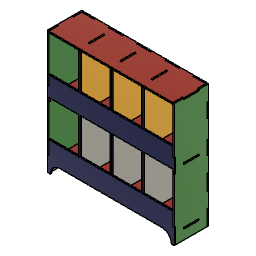
sorted_smarties_collector_finger_joints (Autodesk Fusion 360 design; units mm, degrees)
Autodesk Fusion 360 part; units mm, degrees
note: some values were not read from the file. Chosen so that the rebuilt part matches the saved one: which bodies a step acts on; which face or edge a step refers to; that a step has no effect. Set by a fixed rule: which sketch regions a step uses.
(part 1 of 2)
sketch "Sorted Smarties Collector" plane through (0, 0, 0) normal (0, 1, 0) x (1, 0, 0)
  line L0 (0, 0) -> (266, 0)
  line L1 (266, 0) -> (266, -258)
  line L2 (266, -258) -> (0, -258)
  line L3 (0, -258) -> (0, 0)
  dimension "d1" = 266
  dimension "d41" = 258
  constraint horizontal L0
  constraint vertical L1
  constraint horizontal L2
  constraint vertical L3
  constraint coincident L0.start L3.end
  measures "d1" distance of L0.start L0.end
  measures "d41" distance of L0.end L1.end
extrude "Extrude1" add sketch "Sorted Smarties Collector" along normal blind 3 makes body 1
sketch "Smartie Collectors" plane through (0, 3, 0) normal (0, 1, 0) x (-1, 0, 0)
  line L0 (0, 258) -> (-266, 258)
  line L1 (-266, 258) -> (-266, 0)
  line L2 (-266, 0) -> (0, 0)
  line L3 (0, 0) -> (0, 258)
  line L4 (-263, 255) -> (-200.25, 255)
  line L5 (-200.25, 255) -> (-200.25, 140.5)
  line L6 (-200.25, 140.5) -> (-263, 140.5)
  line L7 (-263, 140.5) -> (-263, 255)
  line L8 (-197.25, 255) -> (-134.5, 255)
  line L9 (-134.5, 255) -> (-134.5, 140.5)
  line L10 (-134.5, 140.5) -> (-197.25, 140.5)
  line L11 (-197.25, 140.5) -> (-197.25, 255)
  line L12 (-131.5, 255) -> (-68.75, 255)
  line L13 (-68.75, 255) -> (-68.75, 140.5)
  line L14 (-68.75, 140.5) -> (-131.5, 140.5)
  line L15 (-131.5, 140.5) -> (-131.5, 255)
  line L16 (-65.75, 255) -> (-3, 255)
  line L17 (-3, 255) -> (-3, 140.5)
  line L18 (-3, 140.5) -> (-65.75, 140.5)
  line L19 (-65.75, 140.5) -> (-65.75, 255)
  line L20 (-263, 137.5) -> (-200.25, 137.5)
  line L21 (-200.25, 137.5) -> (-200.25, 23)
  line L22 (-200.25, 23) -> (-263, 23)
  line L23 (-263, 23) -> (-263, 137.5)
  line L24 (-197.25, 137.5) -> (-134.5, 137.5)
  line L25 (-134.5, 137.5) -> (-134.5, 23)
  line L26 (-134.5, 23) -> (-197.25, 23)
  line L27 (-197.25, 23) -> (-197.25, 137.5)
  line L28 (-131.5, 137.5) -> (-68.75, 137.5)
  line L29 (-68.75, 137.5) -> (-68.75, 23)
  line L30 (-68.75, 23) -> (-131.5, 23)
  line L31 (-131.5, 23) -> (-131.5, 137.5)
  line L32 (-65.75, 137.5) -> (-3, 137.5)
  line L33 (-3, 137.5) -> (-3, 23)
  line L34 (-3, 23) -> (-65.75, 23)
  line L35 (-65.75, 23) -> (-65.75, 137.5)
  line L36 (-263, 0) -> (-3, 0)
  line L37 (-3, 0) -> (-3, 20)
  line L38 (-3, 20) -> (-263, 20)
  line L39 (-263, 20) -> (-263, 0)
  dimension "d51" = 3
  dimension "d52" = 3
  dimension "d53" = 3
  dimension "d54" = 20
  dimension "d55" = 3
  dimension "d56" = 3
  dimension "d57" = 3
  dimension "d58" = 3
  dimension "d59" = 3
  dimension "d60" = 114.5
  dimension "d61" = 114.5
  dimension "d62" = 62.75
  dimension "d63" = 62.75
  dimension "d64" = 62.75
  dimension "d65" = 62.75
  constraint horizontal L4
  constraint vertical L5
  constraint horizontal L6
  constraint vertical L7
  constraint horizontal L8
  constraint vertical L9
  constraint horizontal L10
  constraint vertical L11
  constraint horizontal L12
  constraint vertical L13
  constraint horizontal L14
  constraint vertical L15
  constraint horizontal L16
  constraint vertical L17
  constraint horizontal L18
  constraint vertical L19
  constraint horizontal L20
  constraint vertical L21
  constraint horizontal L22
  constraint vertical L23
  constraint horizontal L24
  constraint vertical L25
  constraint horizontal L26
  constraint vertical L27
  constraint horizontal L28
  constraint vertical L29
  constraint horizontal L30
  constraint vertical L31
  constraint horizontal L32
  constraint vertical L33
  constraint horizontal L34
  constraint vertical L35
  constraint collinear L4 L8
  constraint collinear L8 L12
  constraint collinear L12 L16
  constraint collinear L6 L10
  constraint collinear L10 L14
  constraint collinear L14 L18
  constraint collinear L22 L26
  constraint collinear L26 L30
  constraint collinear L30 L34
  constraint collinear L20 L24
  constraint collinear L24 L28
  constraint collinear L28 L32
  constraint horizontal L36
  constraint vertical L37
  constraint horizontal L38
  constraint vertical L39
  constraint coincident L2 L36.start
  constraint collinear L23 L39
  constraint collinear L7 L23
  constraint collinear L5 L21
  constraint collinear L11 L27
  constraint collinear L9 L25
  constraint collinear L15 L31
  constraint collinear L13 L29
  constraint collinear L19 L35
  constraint collinear L17 L33
  constraint collinear L33 L37
  measures "d51" distance of L0 L4
  measures "d52" distance of L6 L20
  measures "d53" distance of L22 L38
  measures "d54" distance of L36 L38
  measures "d55" distance of L5 L11
  measures "d56" distance of L9 L15
  measures "d57" distance of L13 L19
  measures "d58" distance of L1 L7
  measures "d59" distance of L3 L17
  measures "d60" distance of L16.end L17.end
  measures "d61" distance of L32.end L33.end
  measures "d62" distance of L4.start L4.end
  measures "d63" distance of L8.start L8.end
  measures "d64" distance of L12.start L12.end
  measures "d65" distance of L16.start L16.end
extrude "Extrude2" add sketch "Smartie Collectors" along normal blind 69 contours L0 L1 L2 L3 L37 L38 L39 bodies 1
sketch "Front Panel" plane through (266, 0, 0) normal (1, 0, 0) x (0, 1, 0)
  line L0 (0, 258) -> (0, 0)
  line L1 (0, 0) -> (72, 0)
  line L2 (72, 0) -> (72, 258)
  line L3 (72, 258) -> (0, 258)
  line L4 (72, 258) -> (69, 258)
  line L5 (69, 258) -> (69, 0)
  line L6 (69, 0) -> (72, 0)
  line L7 (72, 0) -> (72, 258)
  dimension "d66" = 3
  constraint horizontal L4
  constraint vertical L5
  constraint horizontal L6
  constraint vertical L7
  constraint coincident L1 L5.end
  constraint coincident L2.end L3.start
  measures "d66" distance of L5.end L1.end
extrude "Extrude3" add sketch "Front Panel" against normal blind 266 contours L1 L2 L3 L4 L5 L6 L7 bodies 1
sketch "Front Openings" plane through (0, 72, 0) normal (0, 1, 0) x (-1, 0, 0)
  line L0 (-266, 0) -> (0, 0)
  line L1 (0, 0) -> (0, 258)
  line L2 (0, 258) -> (-266, 258)
  line L3 (-266, 258) -> (-266, 0)
  line L4 (0, 258) -> (-266, 258)
  line L5 (-197.25, 255) -> (-134.5, 255)
  line L6 (-263, 255) -> (-200.25, 255)
  line L7 (-200.25, 140.5) -> (-263, 140.5)
  line L8 (-263, 137.5) -> (-200.25, 137.5)
  line L9 (-200.25, 23) -> (-263, 23)
  line L10 (-134.5, 23) -> (-197.25, 23)
  line L11 (-68.75, 23) -> (-131.5, 23)
  line L12 (-3, 23) -> (-65.75, 23)
  line L13 (-131.5, 137.5) -> (-68.75, 137.5)
  line L14 (-197.25, 137.5) -> (-134.5, 137.5)
  line L15 (-134.5, 140.5) -> (-197.25, 140.5)
  line L16 (-68.75, 140.5) -> (-131.5, 140.5)
  line L17 (-3, 140.5) -> (-65.75, 140.5)
  line L18 (-65.75, 137.5) -> (-3, 137.5)
  line L19 (-131.5, 255) -> (-68.75, 255)
  line L20 (-65.75, 255) -> (-3, 255)
  line L21 (-3, 20) -> (-263, 20)
  line L22 (-3, 0) -> (-3, 20)
  line L23 (-263, 20) -> (-263, 0)
  line L24 (-263, 23) -> (-263, 137.5)
  line L25 (-200.25, 137.5) -> (-200.25, 23)
  line L26 (-197.25, 23) -> (-197.25, 137.5)
  line L27 (-134.5, 137.5) -> (-134.5, 23)
  line L28 (-131.5, 23) -> (-131.5, 137.5)
  line L29 (-68.75, 137.5) -> (-68.75, 23)
  line L30 (-65.75, 23) -> (-65.75, 137.5)
  line L31 (-3, 137.5) -> (-3, 23)
  line L32 (-263, 140.5) -> (-263, 255)
  line L33 (-200.25, 255) -> (-200.25, 140.5)
  line L34 (-197.25, 140.5) -> (-197.25, 255)
  line L35 (-134.5, 255) -> (-134.5, 140.5)
  line L36 (-131.5, 140.5) -> (-131.5, 255)
  line L37 (-68.75, 255) -> (-68.75, 140.5)
  line L38 (-65.75, 140.5) -> (-65.75, 255)
  line L39 (-3, 255) -> (-3, 140.5)
  line L40 (-263, 255) -> (-200.25, 255)
  line L41 (-200.25, 255) -> (-200.25, 178.6667)
  line L42 (-200.25, 178.6667) -> (-263, 178.6667)
  line L43 (-263, 178.6667) -> (-263, 255)
  line L44 (-197.25, 255) -> (-134.5, 255)
  line L45 (-134.5, 255) -> (-134.5, 178.6667)
  line L46 (-134.5, 178.6667) -> (-197.25, 178.6667)
  line L47 (-197.25, 178.6667) -> (-197.25, 255)
  line L48 (-131.5, 255) -> (-68.75, 255)
  line L49 (-68.75, 255) -> (-68.75, 178.6667)
  line L50 (-68.75, 178.6667) -> (-131.5, 178.6667)
  line L51 (-131.5, 178.6667) -> (-131.5, 255)
  line L52 (-65.75, 255) -> (-3, 255)
  line L53 (-3, 255) -> (-3, 178.6667)
  line L54 (-3, 178.6667) -> (-65.75, 178.6667)
  line L55 (-65.75, 178.6667) -> (-65.75, 255)
  line L56 (-263, 137.5) -> (-200.25, 137.5)
  line L57 (-200.25, 137.5) -> (-200.25, 61.1667)
  line L58 (-200.25, 61.1667) -> (-263, 61.1667)
  line L59 (-263, 61.1667) -> (-263, 137.5)
  line L60 (-197.25, 137.5) -> (-134.5, 137.5)
  line L61 (-134.5, 137.5) -> (-134.5, 61.1667)
  line L62 (-134.5, 61.1667) -> (-197.25, 61.1667)
  line L63 (-197.25, 61.1667) -> (-197.25, 137.5)
  line L64 (-131.5, 137.5) -> (-68.75, 137.5)
  line L65 (-68.75, 137.5) -> (-68.75, 61.1667)
  line L66 (-68.75, 61.1667) -> (-131.5, 61.1667)
  line L67 (-131.5, 61.1667) -> (-131.5, 137.5)
  line L68 (-65.75, 137.5) -> (-3, 137.5)
  line L69 (-3, 137.5) -> (-3, 61.1667)
  line L70 (-3, 61.1667) -> (-65.75, 61.1667)
  line L71 (-65.75, 61.1667) -> (-65.75, 137.5)
  line L72 (-3, 20) -> (-3, 0)
  line L73 (-3, 0) -> (-263, 0)
  line L74 (-263, 0) -> (-263, 20)
  dimension "d72" = 76.3333
  dimension "d73" = 76.3333
  dimension "d84" = 62.75
  dimension "d85" = 62.75
  dimension "d86" = 62.75
  dimension "d87" = 62.75
  dimension "d88" = 62.75
  dimension "d89" = 62.75
  dimension "d90" = 62.75
  dimension "d91" = 62.75
  dimension "d92" = 3
  dimension "d93" = 3
  dimension "d94" = 3
  dimension "d95" = 3
  dimension "d97" = 3
  dimension "d98" = 3
  dimension "d99" = 3
  dimension "d100" = 3
  constraint horizontal L40
  constraint vertical L41
  constraint horizontal L42
  constraint vertical L43
  constraint coincident L6.start L32.end
  constraint horizontal L44
  constraint vertical L45
  constraint horizontal L46
  constraint vertical L47
  constraint coincident L5.start L34.end
  constraint horizontal L48
  constraint vertical L49
  constraint horizontal L50
  constraint vertical L51
  constraint coincident L19.start L36.end
  constraint horizontal L52
  constraint vertical L53
  constraint horizontal L54
  constraint vertical L55
  constraint coincident L20.start L38.end
  constraint horizontal L56
  constraint vertical L57
  constraint horizontal L58
  constraint vertical L59
  constraint coincident L8.start L24.end
  constraint horizontal L60
  constraint vertical L61
  constraint horizontal L62
  constraint vertical L63
  constraint coincident L14.start L26.end
  constraint horizontal L64
  constraint vertical L65
  constraint horizontal L66
  constraint vertical L67
  constraint coincident L13.start L28.end
  constraint horizontal L68
  constraint vertical L69
  constraint horizontal L70
  constraint vertical L71
  constraint coincident L18.start L30.end
  constraint collinear L42 L46
  constraint collinear L46 L50
  constraint collinear L50 L54
  constraint collinear L58 L62
  constraint collinear L62 L66
  constraint collinear L66 L70
  constraint vertical L72
  constraint horizontal L73
  constraint vertical L74
  constraint coincident L22.start L72.end
  constraint coincident L21.end L23.start
  measures "d72" distance of L6.start L42.end
  measures "d73" distance of L8.start L58.end
  measures "d84" distance of L41 L43
  measures "d85" distance of L45 L47
  measures "d86" distance of L49 L51
  measures "d87" distance of L53 L55
  measures "d88" distance of L57 L59
  measures "d89" distance of L61 L63
  measures "d90" distance of L65 L67
  measures "d91" distance of L69 L71
  measures "d92" distance of L3 L43
  measures "d93" distance of L41 L47
  measures "d94" distance of L45 L51
  measures "d95" distance of L49 L55
  measures "d97" distance of L57 L63
  measures "d98" distance of L61 L67
  measures "d99" distance of L65 L71
  measures "d100" distance of L1 L69
extrude "Extrude4" cut sketch "Front Openings" against normal blind 3 contours L5 L34 L35 L44 L45 L46 L47 | L6 L32 L33 L40 L41 L42 L43 | L8 L24 L25 L56 L57 L58 L59 | L14 L26 L27 L60 L61 L62 L63 | L13 L28 L29 L64 L65 L66 L67 | L18 L30 L31 L68 L69 L70 L71 | L19 L36 L37 L48 L49 L50 L51 | L20 L38 L39 L52 L53 L54 L55 bodies 1
sketch "Slide Handle" plane through (0, 0, 0) normal (0, -1, 0) x (1, 0, 0)
  line L0 (0, 258) -> (0, 0)
  line L1 (0, 0) -> (266, 0)
  line L2 (266, 0) -> (266, 258)
  line L3 (3, 20) -> (263, 20)
  line L4 (3, 0) -> (3, 20)
  line L5 (263, 20) -> (263, 0)
  line L6 (263, 0) -> (3, 0)
  line L7 (266, 258) -> (266, 0)
  line L8 (0, 0) -> (0, 258)
  line L9 (0, 258) -> (266, 258)
  line L10 (266, 0) -> (0, 0)
  line L11 (26, 0) -> (240, 0)
  line L12 (240, 0) -> (240, 20)
  line L13 (240, 20) -> (26, 20)
  line L14 (26, 20) -> (26, 0)
  circle A0 centre (26, 0) radius 20
  circle A1 centre (240, 0) radius 20
  point P0 (266, 0)
  dimension "d77" = 20
  dimension "d78" = 40
  dimension "d79" = 40
  dimension "d80" = 26
  dimension "d81" = 26
  constraint horizontal L11
  constraint vertical L12
  constraint horizontal L13
  constraint vertical L14
  constraint coincident L1 L11.start
  constraint coincident L11.start L14.end
  constraint coincident L11.end L12.start
  measures "d77" distance of L11 L13
  measures "d78" diameter of A0
  measures "d79" diameter of A1
  measures "d80" distance of P0 L11.end
  measures "d81" distance of L0.end L11.start
extrude "Extrude5" cut sketch "Slide Handle" against normal blind 72 contours L1 L6 L10 L14 A0 | L1 L6 L10 L11 L14 A0 | L1 L3 L6 L10 L11 L13 A0 A1 | L1 L6 L10 L12 A1 | L1 L6 L10 L11 L12 A1 bodies 1
move_body "Move1" bodies 1 to x (-1, 0, 0) y (0, -1, 0) z (0, 0, 1) at (0, 0, 0)
ref_plane "WorkPlane1" through (-133, -69, 129) normal (0, -1, 0) x (0, 0, 1)
split "Split1" by plane through (-133, -69, 129) normal (0, -1, 0) bodies 1 makes body 2 at (-133.5, -72, 33.7222)
move_body "Move2" bodies 2 to x (1, 0, 0) y (0, 1, 0) z (0, 0, 1) at (0, -80, 0)
ref_plane "WorkPlane2" through (-133, -3, 129) normal (0, 1, 0) x (1, 0, 0)
split "Split2" by plane through (-133, -3, 129) normal (0, 1, 0) bodies 1 makes body 3 at (-97.3333, 0, 178.6667)
move_body "Move3" bodies 3 to x (1, 0, 0) y (0, 1, 0) z (0, 0, 1) at (0, 50, 0)
ref_plane "WorkPlane3" through (-3, -36, 129) normal (1, 0, 0) x (0, 0, 1)
split "Split3" by plane through (-3, -36, 129) normal (1, 0, 0) bodies 1 makes body 4 at (0, -25, 172)
move_body "Move4" bodies 4 to x (1, 0, 0) y (0, 1, 0) z (0, 0, 1) at (80, 0, 0)
ref_plane "WorkPlane4" through (-263, -36, 129) normal (-1, 0, 0) x (0, 0, -1)
split "Split4" by plane through (-263, -36, 129) normal (-1, 0, 0) bodies 1 makes body 5 at (-266, -25, 86)
move_body "Move5" bodies 5 to x (1, 0, 0) y (0, 1, 0) z (0, 0, 1) at (-72, 0, 0)
form "Form1" [no effect]
ref_plane "WorkPlane5" through (-133, -36, 255) normal (0, 0, 1) x (-1, 0, 0)
split "Split5" by plane through (-133, -36, 255) normal (0, 0, 1) bodies 1 makes body 6 at (-176.3333, -47, 258)
move_body "Move6" bodies 6 to x (1, 0, 0) y (0, 1, 0) z (0, 0, 1) at (0, 0, 80)
ref_plane "WorkPlane6" through (-34.375, -36, 140.5) normal (0, 0, 1) x (-1, 0, 0)
split "Split6" by plane through (-34.375, -36, 140.5) normal (0, 0, 1) bodies 1 makes body 7 at (-131.5, -25, 191.3889) makes body 8 at (-197.25, -25, 191.3889) makes body 9 at (-68.75, -25, 191.3889)
ref_plane "WorkPlane7" through (-34.375, -36, 23) normal (0, 0, 1) x (-1, 0, 0)
split "Split7" by plane through (-34.375, -36, 23) normal (0, 0, 1) bodies 1 makes body 10 at (-131.5, -25, 73.8889)
move_body "Move7" bodies 1 to x (1, 0, 0) y (0, 1, 0) z (0, 0, 1) at (0, 0, -80)
sketch "Sketch7" plane through (0, -152, 0) normal (0, -1, 0) x (1, 0, 0)
  arc A0 (-240, 20) -> (-260, 0) centre (-240, 0) ccw
  line L0 (-240, 20) -> (-26, 20)
  arc A1 (-6, 0) -> (-26, 20) centre (-26, 0) ccw
  line L1 (-6, 0) -> (0, 0)
  line L2 (0, 0) -> (0, 258)
  line L3 (0, 258) -> (-266, 258)
  line L4 (-266, 258) -> (-266, 0)
  line L5 (-266, 0) -> (-260, 0)
  line L6 (-200.25, 137.5) -> (-200.25, 61.1667)
  line L7 (-200.25, 61.1667) -> (-263, 61.1667)
  line L8 (-263, 61.1667) -> (-263, 137.5)
  line L9 (-263, 137.5) -> (-200.25, 137.5)
  line L10 (-3, 255) -> (-3, 178.6667)
  line L11 (-3, 178.6667) -> (-65.75, 178.6667)
  line L12 (-65.75, 178.6667) -> (-65.75, 255)
  line L13 (-65.75, 255) -> (-3, 255)
  line L14 (-200.25, 255) -> (-200.25, 178.6667)
  line L15 (-200.25, 178.6667) -> (-263, 178.6667)
  line L16 (-263, 178.6667) -> (-263, 255)
  line L17 (-263, 255) -> (-200.25, 255)
  line L18 (-3, 137.5) -> (-3, 61.1667)
  line L19 (-3, 61.1667) -> (-65.75, 61.1667)
  line L20 (-65.75, 61.1667) -> (-65.75, 137.5)
  line L21 (-65.75, 137.5) -> (-3, 137.5)
  line L22 (-134.5, 137.5) -> (-134.5, 61.1667)
  line L23 (-134.5, 61.1667) -> (-197.25, 61.1667)
  line L24 (-197.25, 61.1667) -> (-197.25, 137.5)
  line L25 (-197.25, 137.5) -> (-134.5, 137.5)
  line L26 (-68.75, 255) -> (-68.75, 178.6667)
  line L27 (-68.75, 178.6667) -> (-131.5, 178.6667)
  line L28 (-131.5, 178.6667) -> (-131.5, 255)
  line L29 (-131.5, 255) -> (-68.75, 255)
  line L30 (-134.5, 255) -> (-134.5, 178.6667)
  line L31 (-134.5, 178.6667) -> (-197.25, 178.6667)
  line L32 (-197.25, 178.6667) -> (-197.25, 255)
  line L33 (-197.25, 255) -> (-134.5, 255)
  line L34 (-68.75, 137.5) -> (-68.75, 61.1667)
  line L35 (-68.75, 61.1667) -> (-131.5, 61.1667)
  line L36 (-131.5, 61.1667) -> (-131.5, 137.5)
  line L37 (-131.5, 137.5) -> (-68.75, 137.5)
sketch "Sketch8" plane through (0, 50, 0) normal (0, 1, 0) x (-1, 0, 0)
  arc A0 (260, 0) -> (240, 20) centre (240, 0) ccw
  line L0 (260, 0) -> (266, 0)
  line L1 (266, 0) -> (266, 258)
  line L2 (266, 258) -> (0, 258)
  line L3 (0, 258) -> (0, 0)
  line L4 (0, 0) -> (6, 0)
  arc A1 (26, 20) -> (6, 0) centre (26, 0) ccw
  line L5 (26, 20) -> (240, 20)
move_body "Move8" bodies 6 to x (1, 0, 0) y (0, 1, 0) z (0, 0, 1) at (0, 0, -80)
move_body "Move9" bodies 3 to x (1, 0, 0) y (0, 1, 0) z (0, 0, 1) at (0, -50, 0)
move_body "Move10" bodies 5 to x (1, 0, 0) y (0, 1, 0) z (0, 0, 1) at (72, 0, 0)
move_body "Move11" bodies 4 to x (1, 0, 0) y (0, 1, 0) z (0, 0, 1) at (-80, 0, 0)
move_body "Move12" bodies 2 to x (1, 0, 0) y (0, 1, 0) z (0, 0, 1) at (0, 80, 0)
move_body "Move13" bodies 1 to x (1, 0, 0) y (0, 1, 0) z (0, 0, 1) at (0, 0, 57)
move_body "Move14" bodies 1 to x (1, 0, 0) y (0, 1, 0) z (0, 0, 1) at (0, 0, 23)
sketch "Sketch9" plane through (0, 0, 0) normal (1, 0, 0) x (0, 1, 0)
  line L0 (-3, 0) -> (-3, 258)
  line L1 (-3, 258) -> (-69, 258)
  line L2 (-69, 258) -> (-69, 0)
  line L3 (-69, 0) -> (-3, 0)
  line L4 (-3, 225.75) -> (-69, 225.75)
  line L5 (-3, 193.5) -> (-69, 193.5)
  line L6 (-3, 161.25) -> (-69, 161.25)
  line L7 (-3, 129) -> (-69, 129)
  line L8 (-3, 96.75) -> (-69, 96.75)
  line L9 (-3, 64.5) -> (-69, 64.5)
  line L10 (-3, 32.25) -> (-69, 32.25)
  line L11 (-69, 225.75) -> (0, 225.75)
  line L12 (0, 225.75) -> (-72, 225.75)
  line L13 (-3, 258) -> (0, 258)
  line L14 (0, 258) -> (0, 225.75)
  line L15 (0, 225.75) -> (-3, 225.75)
  line L16 (-3, 225.75) -> (-3, 258)
  line L17 (-72, 225.75) -> (-69, 225.75)
  line L18 (-69, 225.75) -> (-69, 258)
  line L19 (-69, 258) -> (-72, 258)
  line L20 (-72, 258) -> (-72, 225.75)
  line L21 (-3, 193.5) -> (-69, 193.5)
  line L22 (-69, 193.5) -> (-69, 161.25)
  line L23 (-69, 161.25) -> (-3, 161.25)
  line L24 (-3, 161.25) -> (-3, 193.5)
  line L25 (-72, 158.25) -> (0, 158.25)
  line L26 (0, 158.25) -> (0, 196.5)
  line L27 (0, 196.5) -> (-72, 196.5)
  line L28 (-72, 196.5) -> (-72, 158.25)
  line L29 (0, 225.75) -> (-3, 225.75)
  line L30 (-3, 225.75) -> (-3, 196.5)
  line L31 (-3, 196.5) -> (0, 196.5)
  line L32 (0, 196.5) -> (0, 225.75)
  line L33 (-72, 225.75) -> (-69, 225.75)
  line L34 (-69, 225.75) -> (-69, 196.5)
  line L35 (-69, 196.5) -> (-72, 196.5)
  line L36 (-72, 196.5) -> (-72, 225.75)
  line L37 (0, 158.25) -> (-3, 158.25)
  line L38 (-3, 158.25) -> (-3, 129)
  line L39 (-3, 129) -> (0, 129)
  line L40 (0, 129) -> (0, 158.25)
  line L41 (-72, 158.25) -> (-69, 158.25)
  line L42 (-69, 158.25) -> (-69, 129)
  line L43 (-69, 129) -> (-72, 129)
  line L44 (-72, 129) -> (-72, 158.25)
  line L45 (0, 129) -> (-3, 129)
  line L46 (-3, 129) -> (-3, 96.75)
  line L47 (-3, 96.75) -> (0, 96.75)
  line L48 (0, 96.75) -> (0, 129)
  line L49 (-72, 129) -> (-69, 129)
  line L50 (-69, 129) -> (-69, 96.75)
  line L51 (-69, 96.75) -> (-72, 96.75)
  line L52 (-72, 96.75) -> (-72, 129)
  line L53 (-72, 96.75) -> (-69, 96.75)
  line L54 (-69, 96.75) -> (-69, 64.5)
  line L55 (-69, 64.5) -> (-72, 64.5)
  line L56 (-72, 64.5) -> (-72, 96.75)
  line L57 (-72, 64.5) -> (-69, 64.5)
  line L58 (-69, 64.5) -> (-69, 32.25)
  line L59 (-69, 32.25) -> (-72, 32.25)
  line L60 (-72, 32.25) -> (-72, 64.5)
  line L61 (-69, 0) -> (-72, 0)
  line L62 (-72, 0) -> (-72, 32.25)
  line L63 (-72, 32.25) -> (-69, 32.25)
  line L64 (-69, 32.25) -> (-69, 0)
  line L65 (0, 0) -> (-3, 0)
  line L66 (-3, 0) -> (-3, 32.25)
  line L67 (-3, 32.25) -> (0, 32.25)
  line L68 (0, 32.25) -> (0, 0)
  line L69 (0, 96.75) -> (-3, 96.75)
  line L70 (-3, 96.75) -> (-3, 64.5)
  line L71 (-3, 64.5) -> (0, 64.5)
  line L72 (0, 64.5) -> (0, 96.75)
  line L73 (0, 64.5) -> (-3, 64.5)
  line L74 (-3, 64.5) -> (-3, 32.25)
  line L75 (-3, 32.25) -> (0, 32.25)
  line L76 (0, 32.25) -> (0, 64.5)
  dimension "d108" = -32.25
  dimension "d109" = -64.5
  dimension "d110" = -96.75
  dimension "d111" = -129
  dimension "d112" = -161.25
  dimension "d113" = -193.5
  dimension "d114" = -225.75
  dimension "d115" = 72
  dimension "d116" = 3
  constraint perpendicular L2 L11
  constraint perpendicular L2 L12
  constraint horizontal L13
  constraint vertical L14
  constraint horizontal L15
  constraint vertical L16
  constraint coincident L0.end L1.start
  constraint horizontal L17
  constraint vertical L18
  constraint horizontal L19
  constraint vertical L20
  constraint coincident L1.end L2.start
  constraint horizontal L21
  constraint vertical L22
  constraint horizontal L23
  constraint vertical L24
  constraint horizontal L29
  constraint vertical L30
  constraint horizontal L31
  constraint vertical L32
  constraint coincident L27 L30.end
  constraint coincident L0 L30.end
  constraint horizontal L33
  constraint vertical L34
  constraint horizontal L35
  constraint vertical L36
  constraint coincident L27 L34.end
  constraint coincident L2 L34.end
  constraint horizontal L37
  constraint vertical L38
  constraint horizontal L39
  constraint vertical L40
  constraint horizontal L41
  constraint vertical L42
  constraint horizontal L43
  constraint vertical L44
  constraint horizontal L45
  constraint vertical L46
  constraint horizontal L47
  constraint vertical L48
  constraint horizontal L49
  constraint vertical L50
  constraint horizontal L51
  constraint vertical L52
  constraint horizontal L53
  constraint vertical L54
  constraint horizontal L55
  constraint vertical L56
  constraint horizontal L57
  constraint vertical L58
  constraint horizontal L59
  constraint vertical L60
  constraint horizontal L61
  constraint vertical L62
  constraint horizontal L63
  constraint vertical L64
  constraint coincident L2.end L3.start
  constraint horizontal L65
  constraint vertical L66
  constraint horizontal L67
  constraint vertical L68
  constraint coincident L65.start L68.end
  constraint horizontal L69
  constraint vertical L70
  constraint horizontal L71
  constraint vertical L72
  constraint horizontal L73
  constraint vertical L74
  constraint horizontal L75
  constraint vertical L76
  measures "d115" distance of L11.end L12.end
extrude "Extrude6" cut sketch "Sketch9" against normal blind 3 contours L0 L11 L12 L13 L14 L15 L16 L29 | L2 L12 L17 L18 L19 L20 L33 bodies 2 3
extrude "Extrude7" cut sketch "Sketch9" against normal blind 3 contours L0 L24 L25 L26 L27 L31 L37 | L2 L22 L25 L27 L28 L35 L41 bodies 2 3 makes body 11 at (-2, -72, 206.25)
extrude "Extrude8" cut sketch "Sketch9" against normal blind 3 contours L0 L39 L45 L46 L47 L48 L69 | L2 L43 L49 L50 L51 L52 L53 bodies 2 3
extrude "Extrude9" cut sketch "Sketch9" against normal blind 3 contours L0 L67 L71 L73 L74 L75 L76 | L2 L55 L57 L58 L59 L60 L63 bodies 2 3 makes body 12 at (0, -70, 86)
sketch "Sketch10" plane through (0, 0, 0) normal (0, 1, 0) x (-1, 0, 0)
  line L0 (3, 32.25) -> (0, 32.25)
  line L1 (0, 32.25) -> (0, 0)
  line L2 (0, 0) -> (6, 0)
  arc A0 (26, 20) -> (6, 0) centre (26, 0) ccw
  line L3 (26, 20) -> (240, 20)
  arc A1 (260, 0) -> (240, 20) centre (240, 0) ccw
  line L4 (260, 0) -> (266, 0)
  line L5 (266, 0) -> (266, 258)
  line L6 (266, 258) -> (3, 258)
  line L7 (3, 258) -> (3, 225.75)
  line L8 (3, 225.75) -> (0, 225.75)
  line L9 (0, 225.75) -> (0, 196.5)
  line L10 (0, 196.5) -> (3, 196.5)
  line L11 (3, 196.5) -> (3, 158.25)
  line L12 (3, 158.25) -> (0, 158.25)
  line L13 (0, 158.25) -> (0, 129)
  line L14 (0, 129) -> (3, 129)
  line L15 (3, 129) -> (3, 96.75)
  line L16 (3, 96.75) -> (0, 96.75)
  line L17 (0, 96.75) -> (0, 64.5)
  line L18 (0, 64.5) -> (3, 64.5)
  line L19 (3, 64.5) -> (3, 32.25)
  line L20 (0, 64.5) -> (3, 64.5)
  line L21 (3, 64.5) -> (3, 32.25)
  line L22 (3, 32.25) -> (0, 32.25)
  line L23 (0, 32.25) -> (0, 64.5)
  line L24 (0, 129) -> (3, 129)
  line L25 (3, 129) -> (3, 96.75)
  line L26 (3, 96.75) -> (0, 96.75)
  line L27 (0, 96.75) -> (0, 129)
  line L28 (0, 196.5) -> (3, 196.5)
  line L29 (3, 196.5) -> (3, 158.25)
  line L30 (3, 158.25) -> (0, 158.25)
  line L31 (0, 158.25) -> (0, 196.5)
  line L32 (0, 225.75) -> (3, 225.75)
  line L33 (3, 225.75) -> (3, 258)
  line L34 (3, 258) -> (0, 258)
  line L35 (0, 258) -> (0, 225.75)
  constraint horizontal L20
  constraint vertical L21
  constraint horizontal L22
  constraint vertical L23
  constraint coincident L0.start L19.end
  constraint coincident L17.end L18.start
  constraint horizontal L24
  constraint vertical L25
  constraint horizontal L26
  constraint vertical L27
  constraint coincident L15.end L16.start
  constraint coincident L13.end L14.start
  constraint horizontal L28
  constraint vertical L29
  constraint horizontal L30
  constraint vertical L31
  constraint coincident L11.end L12.start
  constraint coincident L9.end L10.start
  constraint horizontal L32
  constraint vertical L33
  constraint horizontal L34
  constraint vertical L35
  constraint coincident L6.end L7.start
  constraint coincident L8.end L9.start
extrude "Extrude10" add sketch "Sketch10" against normal blind 3 separate body contours L0 L18 L19 L20 L21 L22 L23 | L14 L15 L16 L24 L25 L26 L27 | L10 L11 L12 L28 L29 L30 L31 | L7 L8 L32 L33 L34 L35 makes body 13 at (0, -1, 171) makes body 14 at (-3, -2, 118.25) makes body 15 at (0, -2, 247.25) makes body 16 at (0, -2, 43)
combine "Combine1" operation add target body 4 tool bodies 13 14 15 16
sketch "Sketch11" plane through (0, 0, 0) normal (1, 0, 0) x (0, 1, 0)
  line L0 (0, 258) -> (-69, 258)
  line L1 (-69, 258) -> (-69, 0)
  line L2 (-69, 0) -> (-3, 0)
  line L3 (-3, 0) -> (-3, 32.25)
  line L4 (-3, 32.25) -> (0, 32.25)
  line L5 (0, 32.25) -> (0, 64.5)
  line L6 (0, 64.5) -> (-3, 64.5)
  line L7 (-3, 64.5) -> (-3, 96.75)
  line L8 (-3, 96.75) -> (0, 96.75)
  line L9 (0, 96.75) -> (0, 129)
  line L10 (0, 129) -> (-3, 129)
  line L11 (-3, 129) -> (-3, 158.25)
  line L12 (-3, 158.25) -> (0, 158.25)
  line L13 (0, 158.25) -> (0, 196.5)
  line L14 (0, 196.5) -> (-3, 196.5)
  line L15 (-3, 196.5) -> (-3, 225.75)
  line L16 (-3, 225.75) -> (0, 225.75)
  line L17 (0, 225.75) -> (0, 258)
extrude "Extrude11" add sketch "Sketch9" against normal blind 3 separate body contours L2 L55 L57 L58 L59 L60 L63 | L2 L43 L49 L50 L51 L52 L53 | L2 L22 L25 L27 L28 L35 L41 | L2 L12 L17 L18 L19 L20 L33 makes body 17 at (-1, -72, 183.75) makes body 18 at (-1, -69, 118.25) makes body 19 at (-2, -69, 247.25) makes body 20 at (-2, -69, 53.75)
combine "Combine2" operation add target body 17 tool bodies 19 20 18 4
combine "Combine3" operation add target body 11 tool bodies 12 17
sketch "Sketch12" plane through (0, 0, 0) normal (1, 0, 0) x (0, 1, 0)
  line L0 (-72, 258) -> (-72, 158.25)
  line L1 (-72, 158.25) -> (-69, 158.25)
  line L2 (-69, 158.25) -> (-69, 129)
  line L3 (-69, 129) -> (-72, 129)
  line L4 (-72, 129) -> (-72, 32.25)
  line L5 (-72, 32.25) -> (-69, 32.25)
  line L6 (-69, 32.25) -> (-69, 0)
  line L7 (-69, 0) -> (-3, 0)
  line L8 (-3, 0) -> (-3, 32.25)
  line L9 (-3, 32.25) -> (0, 32.25)
  line L10 (0, 32.25) -> (0, 64.5)
  line L11 (0, 64.5) -> (-3, 64.5)
  line L12 (-3, 64.5) -> (-3, 96.75)
  line L13 (-3, 96.75) -> (0, 96.75)
  line L14 (0, 96.75) -> (0, 129)
  line L15 (0, 129) -> (-3, 129)
  line L16 (-3, 129) -> (-3, 158.25)
  line L17 (-3, 158.25) -> (0, 158.25)
  line L18 (0, 158.25) -> (0, 196.5)
  line L19 (0, 196.5) -> (-3, 196.5)
  line L20 (-3, 196.5) -> (-3, 225.75)
  line L21 (-3, 225.75) -> (0, 225.75)
  line L22 (0, 225.75) -> (0, 258)
  line L23 (0, 258) -> (-72, 258)
  line L24 (0, 255) -> (-72, 255)
  line L25 (-36, 258) -> (-52, 258)
  line L26 (-36, 255) -> (-20, 255)
  line L27 (-52, 258) -> (-20, 258)
  line L28 (-20, 258) -> (-20, 255)
  line L29 (-20, 255) -> (-52, 255)
  line L30 (-52, 255) -> (-52, 258)
  dimension "d129" = -3
  dimension "d130" = 16
  dimension "d131" = 16
  constraint midpoint L23 L25.start
  constraint perpendicular L0 L25
  constraint midpoint L24 L26.start
  constraint parallel L24 L26
  constraint horizontal L27
  constraint vertical L28
  constraint horizontal L29
  constraint vertical L30
  measures "d130" distance of L25.start L25.end
  measures "d131" distance of L26.start L26.end
extrude "Extrude12" cut sketch "Sketch12" against normal blind 3 contours L23 L24 L25 L26 L27 L28 L29 L30 bodies 11
extrude "Extrude13" add 1 faces at (-1, -30.6667, 255) along direction (0, 0, 1) blind 3 separate body on bodies 11 makes body 21
combine "Combine4" operation add target body 6 tool bodies 21
sketch "Sketch13" plane through (0, 0, 0) normal (0, 1, 0) x (-1, 0, 0)
  line L0 (3, 32.25) -> (0, 32.25)
  line L1 (0, 32.25) -> (0, 0)
  line L2 (0, 0) -> (6, 0)
  arc A0 (26, 20) -> (6, 0) centre (26, 0) ccw
  line L3 (26, 20) -> (240, 20)
  arc A1 (260, 0) -> (240, 20) centre (240, 0) ccw
  line L4 (260, 0) -> (266, 0)
  line L5 (266, 0) -> (266, 258)
  line L6 (266, 258) -> (3, 258)
  line L7 (3, 258) -> (3, 225.75)
  line L8 (3, 225.75) -> (0, 225.75)
  line L9 (0, 225.75) -> (0, 196.5)
  line L10 (0, 196.5) -> (3, 196.5)
  line L11 (3, 196.5) -> (3, 158.25)
  line L12 (3, 158.25) -> (0, 158.25)
  line L13 (0, 158.25) -> (0, 129)
  line L14 (0, 129) -> (3, 129)
  line L15 (3, 129) -> (3, 96.75)
  line L16 (3, 96.75) -> (0, 96.75)
  line L17 (0, 96.75) -> (0, 64.5)
  line L18 (0, 64.5) -> (3, 64.5)
  line L19 (3, 64.5) -> (3, 32.25)
  line L20 (266, 258) -> (236.45, 258)
  line L21 (236.45, 258) -> (206.9, 258)
  line L22 (206.9, 258) -> (177.35, 258)
  line L23 (177.35, 258) -> (147.8, 258)
  line L24 (147.8, 258) -> (118.25, 258)
  line L25 (118.25, 258) -> (88.7, 258)
  line L26 (88.7, 258) -> (59.15, 258)
  line L27 (59.15, 258) -> (29.6, 258)
  line L28 (29.6, 258) -> (0.05, 258)
  line L29 (266, 255) -> (236.45, 255)
  line L30 (236.45, 255) -> (206.9, 255)
  line L31 (206.9, 255) -> (177.35, 255)
  line L32 (177.35, 255) -> (147.8, 255)
  line L33 (147.8, 255) -> (118.25, 255)
  line L34 (118.25, 255) -> (88.7, 255)
  line L35 (88.7, 255) -> (59.15, 255)
  line L36 (59.15, 255) -> (29.6, 255)
  line L37 (29.6, 255) -> (0.05, 255)
  line L38 (236.45, 255) -> (266, 255)
  line L39 (266, 255) -> (266, 258)
  line L40 (266, 258) -> (236.45, 258)
  line L41 (236.45, 258) -> (236.45, 255)
  line L42 (236.45, 258) -> (206.9, 258)
  line L43 (206.9, 258) -> (206.9, 255)
  line L44 (206.9, 255) -> (236.45, 255)
  line L45 (236.45, 255) -> (236.45, 258)
  line L46 (177.35, 255) -> (206.9, 255)
  line L47 (206.9, 255) -> (206.9, 258)
  line L48 (206.9, 258) -> (177.35, 258)
  line L49 (177.35, 258) -> (177.35, 255)
  line L50 (147.8, 255) -> (177.35, 255)
  line L51 (177.35, 255) -> (177.35, 258)
  line L52 (177.35, 258) -> (147.8, 258)
  line L53 (147.8, 258) -> (147.8, 255)
  line L54 (118.25, 255) -> (147.8, 255)
  line L55 (147.8, 255) -> (147.8, 258)
  line L56 (147.8, 258) -> (118.25, 258)
  line L57 (118.25, 258) -> (118.25, 255)
  line L58 (88.7, 255) -> (118.25, 255)
  line L59 (118.25, 255) -> (118.25, 258)
  line L60 (118.25, 258) -> (88.7, 258)
  line L61 (88.7, 258) -> (88.7, 255)
  line L62 (59.15, 255) -> (88.7, 255)
  line L63 (88.7, 255) -> (88.7, 258)
  line L64 (88.7, 258) -> (59.15, 258)
  line L65 (59.15, 258) -> (59.15, 255)
  line L66 (29.6, 255) -> (59.15, 255)
  line L67 (59.15, 255) -> (59.15, 258)
  line L68 (59.15, 258) -> (29.6, 258)
  line L69 (29.6, 258) -> (29.6, 255)
  line L70 (29.6, 255) -> (0.05, 255)
  line L71 (0.05, 255) -> (0.05, 258)
  line L72 (0.05, 258) -> (29.6, 258)
  line L73 (29.6, 258) -> (29.6, 255)
  dimension "d136" = 29.55
  dimension "d137" = 29.55
  dimension "d138" = 29.55
  dimension "d139" = 29.55
  dimension "d140" = 29.55
  dimension "d141" = 29.55
  dimension "d142" = 29.55
  dimension "d143" = 29.55
  dimension "d144" = 29.55
  dimension "d145" = -3
  constraint coincident L5.end L6.start
  constraint perpendicular L7 L20
  constraint parallel L6 L21
  constraint perpendicular L7 L22
  constraint parallel L6 L23
  constraint parallel L6 L24
  constraint parallel L6 L25
  constraint parallel L6 L26
  constraint perpendicular L7 L27
  constraint parallel L6 L28
  constraint horizontal L38
  constraint vertical L39
  constraint horizontal L40
  constraint vertical L41
  constraint horizontal L42
  constraint vertical L43
  constraint horizontal L44
  constraint vertical L45
  constraint horizontal L46
  constraint vertical L47
  constraint horizontal L48
  constraint vertical L49
  constraint horizontal L50
  constraint vertical L51
  constraint horizontal L52
  constraint vertical L53
  constraint horizontal L54
  constraint vertical L55
  constraint horizontal L56
  constraint vertical L57
  constraint horizontal L58
  constraint vertical L59
  constraint horizontal L60
  constraint vertical L61
  constraint horizontal L62
  constraint vertical L63
  constraint horizontal L64
  constraint vertical L65
  constraint horizontal L66
  constraint vertical L67
  constraint horizontal L68
  constraint vertical L69
  constraint horizontal L70
  constraint vertical L71
  constraint horizontal L72
  constraint vertical L73
  measures "d136" distance of L5.end L20.end
  measures "d137" distance of L20.end L21.end
  measures "d138" distance of L21.end L22.end
  measures "d139" distance of L22.end L23.end
  measures "d140" distance of L23.end L24.end
  measures "d141" distance of L24.end L25.end
  measures "d142" distance of L25.end L26.end
  measures "d143" distance of L26.end L27.end
  measures "d144" distance of L27.end L28.end
extrude "Extrude14" cut sketch "Sketch13" against normal blind 3 contours L6 L21 L30 L41 L42 L43 L44 L45 L47 | L6 L23 L32 L49 L50 L51 L52 L53 L55 | L6 L25 L34 L57 L58 L59 L60 L61 L63 | L6 L27 L36 L65 L66 L67 L68 L69 L73 bodies 3
extrude "Extrude15" add sketch "Sketch13" against normal blind 3 separate body contours L6 L21 L30 L41 L42 L43 L44 L45 L47 | L6 L23 L32 L49 L50 L51 L52 L53 L55 | L6 L25 L34 L57 L58 L59 L60 L61 L63 | L6 L27 L36 L65 L66 L67 L68 L69 L73 makes body 22 at (-167.5, 0, 256) makes body 23 at (-108.4, 0, 256) makes body 24 at (-226.6, 0, 256) makes body 25 at (-39.45, 0, 257)
combine "Combine5" operation add target body 6 tool bodies 22 23 24 25
sketch "Sketch14" plane through (0, 0, 0) normal (0, 1, 0) x (-1, 0, 0)
  line L0 (118.25, 258) -> (118.25, 255)
  line L1 (118.25, 255) -> (88.7, 255)
  line L2 (88.7, 255) -> (88.7, 258)
  line L3 (88.7, 258) -> (59.15, 258)
  line L4 (59.15, 258) -> (59.15, 255)
  line L5 (59.15, 255) -> (29.6, 255)
  line L6 (29.6, 255) -> (29.6, 258)
  line L7 (29.6, 258) -> (3, 258)
  line L8 (3, 258) -> (3, 225.75)
  line L9 (3, 225.75) -> (0, 225.75)
  line L10 (0, 225.75) -> (0, 196.5)
  line L11 (0, 196.5) -> (3, 196.5)
  line L12 (3, 196.5) -> (3, 158.25)
  line L13 (3, 158.25) -> (0, 158.25)
  line L14 (0, 158.25) -> (0, 129)
  line L15 (0, 129) -> (3, 129)
  line L16 (3, 129) -> (3, 96.75)
  line L17 (3, 96.75) -> (0, 96.75)
  line L18 (0, 96.75) -> (0, 64.5)
  line L19 (0, 64.5) -> (3, 64.5)
  line L20 (3, 64.5) -> (3, 32.25)
  line L21 (3, 32.25) -> (0, 32.25)
  line L22 (0, 32.25) -> (0, 0)
  line L23 (0, 0) -> (6, 0)
  arc A0 (26, 20) -> (6, 0) centre (26, 0) ccw
  line L24 (26, 20) -> (240, 20)
  arc A1 (260, 0) -> (240, 20) centre (240, 0) ccw
  line L25 (260, 0) -> (266, 0)
  line L26 (266, 0) -> (266, 258)
  line L27 (266, 258) -> (236.45, 258)
  line L28 (236.45, 258) -> (236.45, 255)
  line L29 (236.45, 255) -> (206.9, 255)
  line L30 (206.9, 255) -> (206.9, 258)
  line L31 (206.9, 258) -> (177.35, 258)
  line L32 (177.35, 258) -> (177.35, 255)
  line L33 (177.35, 255) -> (147.8, 255)
  line L34 (147.8, 255) -> (147.8, 258)
  line L35 (147.8, 258) -> (118.25, 258)
  line L36 (0, 225.75) -> (266, 225.75)
  line L37 (0, 196.5) -> (266, 196.5)
  line L38 (0, 158.25) -> (266, 158.25)
  line L39 (0, 129) -> (266, 129)
  line L40 (0, 96.75) -> (266, 96.75)
  line L41 (0, 64.5) -> (266, 64.5)
  line L42 (0, 32.25) -> (266, 32.25)
  line L43 (263, 0) -> (263, 258)
  dimension "d150" = -3
  constraint coincident L9.end L10.start
  constraint coincident L26 L36.end
  constraint perpendicular L26 L36
  constraint coincident L10.end L11.start
  constraint coincident L26 L37.end
  constraint perpendicular L26 L37
  constraint coincident L13.end L14.start
  constraint coincident L26 L38.end
  constraint perpendicular L26 L38
  constraint coincident L14.end L15.start
  constraint midpoint L26 L39.end
  constraint coincident L17.end L18.start
  constraint coincident L26 L40.end
  constraint perpendicular L26 L40
  constraint coincident L18.end L19.start
  constraint coincident L26 L41.end
  constraint perpendicular L26 L41
  constraint coincident L21.end L22.start
  constraint perpendicular L26 L42
extrude "Extrude16" cut sketch "Sketch14" against normal blind 3 contours L26 L27 L36 L43 | L26 L37 L38 L43 | L26 L39 L40 L43 | L26 L41 L42 L43 bodies 3
extrude "Extrude17" add 4 faces at (-263, -2, 236.5) (-263, -1, 171) (-263, -2, 107.5) (-263, -2, 43) along direction (-1, 0, 0) blind 3 separate body on bodies 3 makes body 26 at (-265, 0, 107.5) makes body 27 at (-265, 0, 236.5) makes body 28 at (-264, 0, 171) makes body 29 at (-264, 0, 43)
combine "Combine6" operation add target body 5 tool bodies 29 28 27 26
sketch "Sketch15" plane through (0, 0, 258) normal (0, 0, 1) x (-1, 0, 0)
  line L0 (263, 3) -> (263, 69)
  line L1 (263, 69) -> (3, 69)
  line L2 (3, 69) -> (3, 52)
  line L3 (3, 52) -> (0, 52)
  line L4 (0, 52) -> (0, 20)
  line L5 (0, 20) -> (3, 20)
  line L6 (3, 20) -> (3, 3)
  line L7 (3, 3) -> (29.6, 3)
  line L8 (29.6, 3) -> (29.6, 0)
  line L9 (29.6, 0) -> (59.15, 0)
  line L10 (59.15, 0) -> (59.15, 3)
  line L11 (59.15, 3) -> (88.7, 3)
  line L12 (88.7, 3) -> (88.7, 0)
  line L13 (88.7, 0) -> (118.25, 0)
  line L14 (118.25, 0) -> (118.25, 3)
  line L15 (118.25, 3) -> (147.8, 3)
  line L16 (147.8, 3) -> (147.8, 0)
  line L17 (147.8, 0) -> (177.35, 0)
  line L18 (177.35, 0) -> (177.35, 3)
  line L19 (177.35, 3) -> (206.9, 3)
  line L20 (206.9, 3) -> (206.9, 0)
  line L21 (206.9, 0) -> (236.45, 0)
  line L22 (236.45, 0) -> (236.45, 3)
  line L23 (236.45, 3) -> (263, 3)
  line L24 (0, 20) -> (265.9567, 20)
  line L25 (265.9567, 20) -> (0, 20)
  line L26 (0, 20) -> (0, 52)
  line L27 (0, 52) -> (265.9567, 52)
  line L28 (265.9567, 52) -> (265.9567, 20)
  constraint coincident L4.end L5.start
  constraint perpendicular L0 L24
  constraint horizontal L25
  constraint vertical L26
  constraint horizontal L27
  constraint vertical L28
  constraint coincident L3.end L4.start
extrude "Extrude18" cut sketch "Sketch15" against normal blind 3 contours L0 L24 L25 L27 L28 bodies 5
extrude "Extrude19" cut 1 faces at (-265.9567, -41.3333, 257) along direction (-1, 0, 0) blind 2 on bodies 5 bodies 5
extrude "Extrude20" add 1 faces at (-264, -41.3333, 255) along direction (0, 0, 1) blind 3 separate body on bodies 5 makes body 30
combine "Combine7" operation add target body 6 tool bodies 30
ref_plane "WorkPlane8" through (-133, -36, 129) normal (1, 0, 0) x (0, 0, 1)
delete_body "RemoveBody1" bodies 5
mirror "Mirror1" about plane through (-133, -36, 129) normal (1, 0, 0) of bodies 11 makes body 31
move_body "Move15" bodies 31 to x (1, 0, 0) y (0, 1, 0) z (0, 0, 1) at (-20, 0, 0)
ref_plane "WorkPlane9" through (-284.5, -36, 208.125) normal (0, -1, 0) x (0, 0, 1)
ref_plane "WorkPlane10" through (-284.5, -36, 241.875) normal (0, 1, 0) x (1, 0, 0)
split "Split8" by plane through (-284.5, -36, 208.125) normal (0, -1, 0) bodies 31 makes body 32 at (-286, -47, 128)
delete_body "RemoveBody2" bodies 32
mirror "Mirror2" about plane through (-284.5, -36, 208.125) normal (0, -1, 0) of bodies 31 merged
sketch "Sketch16" plane through (-286, 0, 0) normal (-1, 0, 0) x (0, -1, 0)
  line L0 (52, 255) -> (20, 255)
  line L1 (20, 255) -> (20, 258)
  line L2 (20, 258) -> (0, 258)
  line L3 (0, 258) -> (0, 225.75)
  line L4 (0, 225.75) -> (3, 225.75)
  line L5 (3, 225.75) -> (3, 196.5)
  line L6 (3, 196.5) -> (0, 196.5)
  line L7 (0, 196.5) -> (0, 158.25)
  line L8 (0, 158.25) -> (3, 158.25)
  line L9 (3, 158.25) -> (3, 129)
  line L10 (3, 129) -> (0, 129)
  line L11 (0, 129) -> (0, 96.75)
  line L12 (0, 96.75) -> (3, 96.75)
  line L13 (3, 96.75) -> (3, 64.5)
  line L14 (3, 64.5) -> (0, 64.5)
  line L15 (0, 64.5) -> (0, 32.25)
  line L16 (0, 32.25) -> (3, 32.25)
  line L17 (3, 32.25) -> (3, 0)
  line L18 (3, 0) -> (69, 0)
  line L19 (69, 0) -> (69, 32.25)
  line L20 (69, 32.25) -> (72, 32.25)
  line L21 (72, 32.25) -> (72, 64.5)
  line L22 (72, 64.5) -> (69, 64.5)
  line L23 (69, 64.5) -> (69, 96.75)
  line L24 (69, 96.75) -> (72, 96.75)
  line L25 (72, 96.75) -> (72, 129)
  line L26 (72, 129) -> (69, 129)
  line L27 (69, 129) -> (69, 158.25)
  line L28 (69, 158.25) -> (72, 158.25)
  line L29 (72, 158.25) -> (72, 196.5)
  line L30 (72, 196.5) -> (69, 196.5)
  line L31 (69, 196.5) -> (69, 225.75)
  line L32 (69, 225.75) -> (72, 225.75)
  line L33 (72, 225.75) -> (72, 258)
  line L34 (72, 258) -> (52, 258)
  line L35 (52, 258) -> (52, 255)
  line L36 (69, 225.75) -> (69, 258)
  line L37 (69, 258) -> (69, 0)
  line L38 (69, 0) -> (72, 0)
  line L39 (72, 0) -> (72, 258)
  line L40 (72, 258) -> (69, 258)
  line L41 (69, 258) -> (69, 0)
  constraint coincident L31.end L32.start
  constraint coincident L34 L36.end
  constraint perpendicular L34 L36
  constraint coincident L18.end L19.start
  constraint horizontal L38
  constraint vertical L39
  constraint horizontal L40
  constraint vertical L41
  constraint coincident L33.end L34.start
extrude "Extrude21" add sketch "Sketch16" against normal blind 3 separate body contours L30 L31 L32 L37 L39 L41 | L26 L27 L28 L37 L39 L41 | L22 L23 L24 L37 L39 L41 | L19 L20 L37 L38 L39 L41 makes body 33 at (-285, -69, 138.75) makes body 34 at (-284, -72, 75.25) makes body 35 at (-285, -72, 206.25) makes body 36 at (-284, -72, 10.75)
move_body "Move16" bodies 33 36 35 34 to x (1, 0, 0) y (0, 1, 0) z (0, 0, 1) at (17, 0, 0)
move_body "Move17" bodies 31 to x (1, 0, 0) y (0, 1, 0) z (0, 0, 1) at (17, 0, 0)
move_body "Move18" bodies 31 to x (1, 0, 0) y (0, 1, 0) z (0, 0, 1) at (-20, 0, 0)
sketch "Sketch17" plane through (-286, 0, 0) normal (1, 0, 0) x (0, 1, 0)
  line L0 (-69, 0) -> (-3, 0)
  line L1 (-3, 0) -> (-3, 32.25)
  line L2 (-3, 32.25) -> (0, 32.25)
  line L3 (0, 32.25) -> (0, 64.5)
  line L4 (0, 64.5) -> (-3, 64.5)
  line L5 (-3, 64.5) -> (-3, 96.75)
  line L6 (-3, 96.75) -> (0, 96.75)
  line L7 (0, 96.75) -> (0, 129)
  line L8 (0, 129) -> (-3, 129)
  line L9 (-3, 129) -> (-3, 158.25)
  line L10 (-3, 158.25) -> (0, 158.25)
  line L11 (0, 158.25) -> (0, 196.5)
  line L12 (0, 196.5) -> (-3, 196.5)
  line L13 (-3, 196.5) -> (-3, 225.75)
  line L14 (-3, 225.75) -> (0, 225.75)
  line L15 (0, 225.75) -> (0, 258)
  line L16 (0, 258) -> (-20, 258)
  line L17 (-20, 258) -> (-20, 255)
  line L18 (-20, 255) -> (-52, 255)
  line L19 (-52, 255) -> (-52, 258)
  line L20 (-52, 258) -> (-72, 258)
  line L21 (-72, 258) -> (-72, 225.75)
  line L22 (-72, 225.75) -> (-69, 225.75)
  line L23 (-69, 225.75) -> (-69, 196.5)
  line L24 (-69, 196.5) -> (-72, 196.5)
  line L25 (-72, 196.5) -> (-72, 158.25)
  line L26 (-72, 158.25) -> (-69, 158.25)
  line L27 (-69, 158.25) -> (-69, 129)
  line L28 (-69, 129) -> (-72, 129)
  line L29 (-72, 129) -> (-72, 96.75)
  line L30 (-72, 96.75) -> (-69, 96.75)
  line L31 (-69, 96.75) -> (-69, 64.5)
  line L32 (-69, 64.5) -> (-72, 64.5)
  line L33 (-72, 64.5) -> (-72, 32.25)
  line L34 (-72, 32.25) -> (-69, 32.25)
  line L35 (-69, 32.25) -> (-69, 0)
  line L36 (-69, 225.75) -> (-69, 265.6091)
  line L37 (-69, 258) -> (-69, -28.5446)
  constraint coincident L22.end L23.start
  constraint perpendicular L22 L36
  constraint coincident L20 L37.start
  constraint coincident L36 L37.start
  constraint perpendicular L20 L37
delete_body "RemoveBody3" bodies 36
delete_body "RemoveBody4" bodies 35
delete_body "RemoveBody5" bodies 34
delete_body "RemoveBody6" bodies 33
mirror "Mirror3" about plane through (-133, -36, 129) normal (1, 0, 0) of bodies 11 makes body 37
move_body "Move19" bodies 37 to x (1, 0, 0) y (0, 1, 0) z (0, 0, 1) at (-120, 0, 0)
delete_body "RemoveBody7" bodies 31
move_body "Move20" bodies 37 to x (1, 0, 0) y (0, 1, 0) z (0, 0, 1) at (117, 0, 0)
move_body "Move21" bodies 37 to x (1, 0, 0) y (0, 1, 0) z (0, 0, 1) at (3, 0, 0)
move_body "Move22" bodies 37 to x (1, 0, 0) y (0, 1, 0) z (0, 0, 1) at (-10, 0, 0)
extrude "Extrude22" add 1 faces at (-275, -69, 138.75) along direction (0, -1, 0) blind 3 separate body on bodies 37 makes body 38
move_body "Move23" bodies 38 to x (1, 0, 0) y (0, 1, 0) z (0, 0, 1) at (7, 0, 0)
extrude "Extrude23" add 1 faces at (-275, -69, 21.5) along direction (0, -1, 0) blind 3 separate body on bodies 37 makes body 39
move_body "Move24" bodies 39 to x (1, 0, 0) y (0, 1, 0) z (0, 0, 1) at (7, 0, 0)
combine "Combine9" operation add target body 2 tool bodies 38 39
extrude "Extrude24" add 1 faces at (-263, -71, 204.1111) along direction (1, 0, 0) blind 3 separate body on bodies 2 makes body 40
extrude "Extrude25" cut 1 faces at (-263, -71, 204.1111) along direction (-1, 0, 0) blind 3 on bodies 2 bodies 2
move_body "Move25" bodies 40 to x (1, 0, 0) y (0, 1, 0) z (0, 0, 1) at (-3, 0, 0)
extrude "Extrude26" add 1 faces at (-266, -70, 64.5) along direction (-1, 0, 0) blind 3 separate body on bodies 2 makes body 41
extrude "Extrude27" cut 1 faces at (-266, -70, 64.5) along direction (1, 0, 0) blind 3 on bodies 2 bodies 2
move_body "Move26" bodies 37 to x (1, 0, 0) y (0, 1, 0) z (0, 0, 1) at (7, 0, 0)
move_body "Move27" bodies 37 to x (1, 0, 0) y (0, 1, 0) z (0, 0, 1) at (3, 0, 0)
extrude "Extrude28" cut 1 faces at (-269, -71, 148.5) along direction (1, 0, 0) blind 3 on bodies 2 bodies 2
extrude "Extrude29" cut 1 faces at (-269, -70, 10.75) along direction (1, 0, 0) blind 3 on bodies 2 bodies 2
move_body "Move28" bodies 2 to x (1, 0, 0) y (0, 1, 0) z (0, 0, 1) at (0, -20, 0)
sketch "Sketch18" plane through (-266, 0, 0) normal (-1, 0, 0) x (0, -1, 0)
  line L0 (92, 178.6667) -> (89, 178.6667)
  line L1 (89, 178.6667) -> (89, 129)
  line L2 (89, 129) -> (92, 129)
  line L3 (92, 129) -> (92, 178.6667)
  line L4 (92, 158.2497) -> (89, 158.2497)
  dimension "d185" = -20.417
extrude "Extrude30" cut sketch "Sketch18" against normal blind 3 contours L0 L1 L3 L4 bodies 2
move_body "Move29" bodies 2 to x (1, 0, 0) y (0, 1, 0) z (0, 0, 1) at (0, 20, 0)
extrude "Extrude31" cut 1 faces at (-266, -71, 256) along direction (1, 0, 0) blind 3 on bodies 2 bodies 2
delete_body "RemoveBody8" bodies 40
delete_body "RemoveBody9" bodies 41
extrude "Extrude32" cut 1 faces at (-263, -71, 256) along direction (-1, 0, 0) blind 3 on bodies 2 bodies 37
move_body "Move30" bodies 2 to x (1, 0, 0) y (0, 1, 0) z (0, 0, 1) at (0, -30, 0)
extrude "Extrude33" add 1 faces at (-263, -101, 256) along direction (-1, 0, 0) blind 3 on bodies 2 bodies 2
move_body "Move31" bodies 2 to x (1, 0, 0) y (0, 1, 0) z (0, 0, 1) at (0, 30, 0)
extrude "Extrude34" add 1 faces at (-89.6667, -69, 256) along direction (0, -1, 0) blind 3 on bodies 6 bodies 6